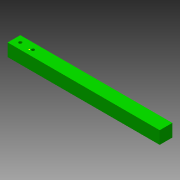
# Autodesk Inventor part: claw arm
Saved by Autodesk Inventor 2015 (Build 190159000, 159)
## iProperties
Created: 2015-01-05
Part Number: claw arm
Material: Generic
Document SubType Name: Modeling
Designer: Collin_2
Density: 1 g/cm^3
Appearance: Default
Author: Collin_2
Autodesk Inventor part; units mm, degrees
ref_plane "YZ Plane" through (0, 0, 0) normal (1, 0, 0) x (0, 1, 0)
ref_plane "XZ Plane" through (0, 0, 0) normal (0, 1, 0) x (-1, 0, 0)
ref_plane "XY Plane" through (0, 0, 0) normal (0, 0, 1) x (1, 0, 0)
sketch "Sketch1" plane through (0, 0, 0) normal (0, 1, 0) x (-1, 0, 0)
  line L0 (68.2659, 18.1219) -> (-541.3341, 18.1219)
  line L1 (-541.3341, 18.1219) -> (-541.3341, -32.6781)
  line L2 (-541.3341, -32.6781) -> (68.2659, -32.6781)
  line L3 (68.2659, -32.6781) -> (68.2659, 18.1219)
  point P0 (0, 0)
  dimension "d0" = 50.8
  dimension "d1" = 609.6
  constraints: 8 end point, 2 parallel, 1 horizontal, 1 perpendicular
  measures "d0" distance of L2.end L0.start
  measures "d1" distance of L1.end L2.end
extrude "Extrusion1" add sketch "Sketch1" along normal blind 50.8
sketch "Sketch2" plane through (0, 50.8, 0) normal (0, 1, 0) x (1, 0, 0)
  line L0 (541.3341, -18.1219) -> (541.3341, 32.6781)
  line L1 (541.3341, -18.1219) -> (541.3341, 32.6781) projected
  line L2 (541.3341, 7.2781) -> (-68.2659, 7.2781)
  circle A0 centre (-42.8659, 7.2781) radius 6.35
  circle A1 centre (7.9341, 7.2781) radius 6.35
  line L3 (-68.2659, 32.6781) -> (-68.2659, -18.1219)
  line L4 (-68.2659, 32.6781) -> (-68.2659, -18.1219) projected
  line L5 (-68.2659, -18.1219) -> (-68.2659, 32.6781)
  point P0 (0, 0)
  dimension "d4" = 12.7
  dimension "d5" = 12.7
  dimension "d8" = 50.8
  dimension "d9" = 25.4
  constraints: 8 end point, 2 centre point, 2 collinear, 2 point on line, 1 horizontal, 1 midpoint
  measures "d4" diameter of A0
  measures "d5" diameter of A1
  measures "d8" distance of A1.centre A0.centre
  measures "d9" distance from line of L3 A0.centre
extrude "Extrusion2" cut sketch "Sketch2" against normal blind 50.8
sketch "Sketch3" plane through (0, 50.8, 0) normal (0, 1, 0) x (1, 0, 0)
  point P0 (0, 0)
body "Solid1"
